Autodesk Fusion 360 part; units mm, degrees
note: some values were not read from the file. Set by a fixed rule: which face or edge a step refers to.
(part 5 of 5)
sketch "Sketch115" plane through (0, 0, 199) normal (0, 0, -1) x (1, 0, 0)
  arc A0 (12.3794, -185.174) -> (17.3688, -190.5) centre (17.3688, -185.5) ccw
  line L0 (17.3688, -190.5) -> (192.6312, -190.5)
  arc A1 (192.6312, -190.5) -> (197.6206, -185.174) centre (192.6312, -185.5) ccw
  line L1 (197.6206, -185.174) -> (187.9915, -37.79)
  line L2 (187.9915, -37.79) -> (186.8719, -35.2665)
  spline S0 degree 3 poles (186.8719, -35.2665) (186.4019, -34.7817) (185.9319, -34.2969) (185.4619, -33.812) (183.1334, -31.4102) (180.2458, -29.0071) (176.8318, -26.5081) (171.496, -22.6022) (164.9221, -18.5059) (158.3928, -15.0439) (153.9573, -12.6921) (149.5874, -10.659) (145.559, -9.2188) (143.1119, -8.3439) (140.848, -7.7157) (138.7248, -7.3463) (137.9673, -7.2145) (137.2067, -7.1126) (136.4309, -7.0548) (135.9483, -7.0188) (135.4719, -7) (135, -7) knots -0.65681 -0.65681 -0.65681 -0.65681 -0.621923 -0.621923 -0.621923 -0.48793 -0.48793 -0.48793 -0.278155 -0.278155 -0.278155 -0.135918 -0.135918 -0.135918 -0.050335 -0.050335 -0.050335 -0.019847 -0.019847 -0.019847 0 0 0 0
  line L3 (135, -7) -> (75, -7)
  spline S1 degree 3 poles (75, -7) (73.2933, -7) (71.6432, -7.2409) (69.934, -7.612) (68.7145, -7.8767) (67.4303, -8.2243) (66.0807, -8.6602) (62.0214, -9.9713) (57.6208, -11.9463) (53.0924, -14.2741) (50.7662, -15.4698) (48.414, -16.7616) (46.1004, -18.1091) (41.0007, -21.0795) (36.1216, -24.2734) (32.0413, -27.3444) (29.1079, -29.5522) (26.6019, -31.6814) (24.5358, -33.8142) (24.0662, -34.299) (23.5966, -34.7837) (23.127, -35.2685) knots 0 0 0 0 0.068385 0.068385 0.068385 0.116327 0.116327 0.116327 0.262353 0.262353 0.262353 0.337245 0.337245 0.337245 0.502934 0.502934 0.502934 0.621914 0.621914 0.621914 0.656812 0.656812 0.656812 0.656812
  line L4 (23.127, -35.2685) -> (22.0085, -37.7909)
  line L5 (22.0085, -37.7909) -> (12.3794, -185.174)
  line L6 (192, -160.5) -> (192, -186.5)
  line L7 (192, -186.5) -> (185, -186.5)
  line L8 (185, -186.5) -> (185, -183)
  line L9 (185, -183) -> (25, -183)
  line L10 (25, -183) -> (25, -186.5)
  line L11 (25, -186.5) -> (18, -186.5)
  line L12 (18, -186.5) -> (18, -160.5)
  line L13 (18, -160.5) -> (26, -160.5)
  line L14 (26, -160.5) -> (26, -38.0516)
  spline S2 degree 3 poles (26, -38.0516) (26.4696, -37.5669) (26.9392, -37.0821) (27.4088, -36.5974) (29.2725, -34.6734) (31.6285, -32.6614) (34.4467, -30.5403) (38.3659, -27.5905) (43.134, -24.4661) (48.1137, -21.5656) (50.3688, -20.252) (52.6617, -18.993) (54.921, -17.8316) (59.3264, -15.5672) (63.5716, -13.6741) (67.3101, -12.4666) (68.5449, -12.0678) (69.7039, -11.7551) (70.7827, -11.5209) (72.3215, -11.1868) (73.6669, -11) (75, -11) knots -0.656812 -0.656812 -0.656812 -0.656812 -0.621914 -0.621914 -0.621914 -0.502934 -0.502934 -0.502934 -0.337245 -0.337245 -0.337245 -0.262353 -0.262353 -0.262353 -0.116327 -0.116327 -0.116327 -0.068385 -0.068385 -0.068385 0 0 0 0
  line L15 (75, -11) -> (135, -11)
  spline S3 degree 3 poles (135, -11) (135.3658, -11) (135.7424, -11.0145) (136.1336, -11.0437) (136.7557, -11.0901) (137.3844, -11.1731) (138.0391, -11.287) (139.8769, -11.6068) (141.9329, -12.1703) (144.2124, -12.9853) (147.9761, -14.3309) (152.2041, -16.29) (156.519, -18.5779) (162.8741, -21.9475) (169.3238, -25.9693) (174.4691, -29.7357) (177.7611, -32.1455) (180.4883, -34.4285) (182.5899, -36.5963) (183.0599, -37.0811) (183.53, -37.5659) (184, -38.0508) knots 0 0 0 0 0.019847 0.019847 0.019847 0.050335 0.050335 0.050335 0.135918 0.135918 0.135918 0.278155 0.278155 0.278155 0.48793 0.48793 0.48793 0.621923 0.621923 0.621923 0.65681 0.65681 0.65681 0.65681
  line L16 (184, -38.0508) -> (184, -160.5)
  line L17 (184, -160.5) -> (192, -160.5)
  line L18 (195.3433, -150.3182) -> (187.3433, -150.3182)
  line L19 (187.3433, -150.3182) -> (187.3433, -149.3182)
  line L20 (187.3433, -149.3182) -> (195.3433, -149.3182)
  line L21 (195.3433, -149.3182) -> (195.3433, -150.3182)
  line L22 (187.3433, -145.0834) -> (195.3433, -145.0834)
  line L23 (195.3433, -145.0834) -> (195.3433, -144.0834)
  line L24 (195.3433, -144.0834) -> (187.3433, -144.0834)
  line L25 (187.3433, -144.0834) -> (187.3433, -145.0834)
  line L26 (194.4182, -182.174) -> (185.0327, -38.5184)
  dimension "d1046" = 8
  dimension "d1047" = 1
  dimension "d1048" = 8
  dimension "d1049" = 1
  constraint horizontal L18
  constraint vertical L19
  constraint horizontal L20
  constraint vertical L21
  constraint coincident L1 L18.start
  constraint horizontal L22
  constraint vertical L23
  constraint horizontal L24
  constraint vertical L25
  measures "d1046" distance of L18.start L18.end
  measures "d1047" distance of L18.start L20.end
  measures "d1048" distance of L22.start L22.end
  measures "d1049" distance of L22.start L24.end
extrude "Extrude63'" cut sketch "Sketch115" against normal blind 2 contours L1 L18 L20 L26 | L1 L22 L24 L26 bodies 28
copy_body "CutPasteBodies3" bodies 28 removing the originals makes body 29 in component "inner_adapter"
sketch "Sketch125" plane through (26, 0, 0) normal (-1, 0, 0) x (0, -1, 0)
  line L0 (-140.5, 125) -> (-140.5, 139)
  line L1 (-140.5, 139) -> (-135.5, 139)
  line L2 (-135.5, 139) -> (-135.5, 125)
  line L3 (-135.5, 125) -> (-38.0516, 125)
  line L4 (-38.0516, 125) -> (-38.0516, 205)
  line L5 (-38.0516, 205) -> (-171.5, 205)
  line L6 (-171.5, 205) -> (-171.5, 133.1623)
  arc A0 (-176.5, 130) -> (-171.5, 133.1623) centre (-173, 130) ccw
  line L7 (-176.5, 130) -> (-176.5, 205)
  line L8 (-176.5, 205) -> (-183, 205)
  line L9 (-183, 205) -> (-183, 125)
  line L10 (-183, 125) -> (-160.5, 125)
  line L11 (-160.5, 125) -> (-160.5, 126.75)
  line L12 (-160.5, 126.75) -> (-157.5, 126.75)
  line L13 (-157.5, 126.75) -> (-157.5, 125)
  line L14 (-157.5, 125) -> (-140.5, 125)
  line L15 (-157.5, 135.25) -> (-157.5, 133.25)
  line L16 (-157.5, 133.25) -> (-162.5, 133.25)
  line L17 (-162.5, 133.25) -> (-162.5, 135.25)
  line L18 (-162.5, 135.25) -> (-157.5, 135.25)
  circle A1 centre (-105.3085, 170) radius 1.5
  line L19 (-151.5, 195) -> (-131.5, 195)
  line L20 (-131.5, 195) -> (-131.5, 153)
  line L21 (-131.5, 153) -> (-151.5, 153)
  line L22 (-151.5, 153) -> (-151.5, 195)
  line L23 (-128.5, 150) -> (-154.5, 150)
  line L24 (-154.5, 150) -> (-154.5, 198)
  line L25 (-154.5, 198) -> (-128.5, 198)
  line L26 (-128.5, 198) -> (-128.5, 150)
  line L27 (-154.5, 150) -> (-147.5, 150)
  line L28 (-147.5, 150) -> (-147.5, 153)
  line L29 (-131.5, 153) -> (-128.5, 153)
  line L30 (-151.5, 153) -> (-151.5, 150)
  line L31 (-151.5, 153) -> (-154.5, 153)
  line L32 (-150.5, 153) -> (-150.5, 194)
  line L33 (-150.5, 194) -> (-132.5, 194)
  line L34 (-132.5, 194) -> (-132.5, 153)
  line L35 (-151.5, 195) -> (-151.5, 190)
  line L36 (-151.5, 153) -> (-151.5, 165)
  line L37 (-151.5, 165) -> (-154.5, 165)
  line L38 (-151.5, 190) -> (-154.5, 190)
  line L39 (-147.5, 153) -> (-147.5, 154.5)
  line L40 (-147.5, 154.5) -> (-151.5, 154.5)
  line L41 (-150.5, 153) -> (-150.5, 150)
  line L42 (-147.5, 151.5) -> (-150.5, 151.5)
  dimension "d1080" = 20
  dimension "d1081" = 42
  dimension "d1082" = 10
  dimension "d1083" = 20
  dimension "d1084" = -3
  dimension "d1085" = 7
  dimension "d1086" = 1
  dimension "d1091" = 5
  dimension "d1092" = 12
  dimension "d1093" = 1.5
  dimension "d1100" = 1.5
  constraint horizontal L19
  constraint vertical L20
  constraint horizontal L21
  constraint vertical L22
  constraint perpendicular L24 L27
  constraint coincident L21 L28.end
  constraint perpendicular L21 L28
  constraint coincident L26 L29.end
  constraint perpendicular L26 L29
  constraint perpendicular L21 L30
  constraint coincident L24 L31.end
  constraint perpendicular L24 L31
  constraint perpendicular L19 L35
  constraint perpendicular L5 L36
  constraint coincident L24 L37.end
  constraint perpendicular L24 L37
  constraint coincident L24 L38.end
  constraint perpendicular L24 L38
  constraint perpendicular L21 L39
  constraint coincident L22 L40.end
  constraint coincident L23 L41.end
  constraint parallel L30 L41
  constraint coincident L28 L42.start
  constraint coincident L41 L42.end
  constraint perpendicular L41 L42
  measures "d1080" distance of L19.start L19.end
  measures "d1081" distance of L19.start L21.end
  measures "d1082" distance of L5 L19
  measures "d1083" distance of L6 L22
  measures "d1085" distance of L23.end L27.end
  measures "d1091" distance of L19.start L35.end
  measures "d1092" distance of L21.end L36.end
  measures "d1093" distance of L28.end L39.end
  measures "d1100" distance of L21 L42
extrude "Extrude64'" add sketch "Sketch125" along normal blind 4 separate body contours L19 L20 L21 L22 L32 L33 L34 L35 L36 L40 | L22 L24 L37 L38 | L21 L23 L26 L28 L29 | L21 L22 L32 L36 L40 | L21 L28 L41 L42 | L21 L23 L27 L30 L41 | L23 L24 L27 L30 L31 | L23 L27 L28 L41 L42 makes body 30
extrude "Extrude65'" add sketch "Sketch125" along normal blind 7 contours L19 L20 L22 L24 L25 L26 L29 L35 L38 | L22 L24 L31 L36 L37 | L21 L28 L41 L42 bodies 30
extrude "Extrude67'" add sketch "Sketch125" along normal blind 1 from surface at 6 contours L21 L32 L39 L40 bodies 30
mirror "Mirror3''" about plane through (105, 109.0383, 160) normal (-1, 0, 0) of bodies 30 makes body 31
copy_body "CutPasteBodies4" bodies 30 31 removing the originals makes body 32 makes body 33 in component "inner_adapter"
component "Outer_Montage_Rim" placed x (1, 0, 0) y (0, 1, 0) z (0, 0, 1) at (0, 0, 0)
component "Tunnel" placed x (1, 0, 0) y (0, 1, 0) z (0, 0, 1) at (0, 0, 0)
component "inner_adapter" placed x (1, 0, 0) y (0, 1, 0) z (0, 0, 1) at (0, 0, 0)
component "Flap" placed x (1, 0, 0) y (0, 1, 0) z (0, 0, 1) at (0, 0, 0)
component "Pins" placed x (1, 0, 0) y (0, 1, 0) z (0, 0, 1) at (0, 0, 0)
component "Mechanism_backstop" placed x (1, 0, 0) y (0, 1, 0) z (0, 0, 1) at (0, 0, 0)
named bodies: "Outer_Montage_Rim", "Tunnel", "RFID_Holder_l", "RFID_Holder_r"
